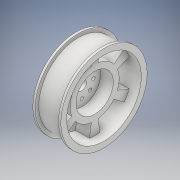
# Autodesk Inventor part: 바퀴8PI
Saved by Autodesk Inventor 2017 (Build 210142000, 142)
## iProperties
Part Number: 바퀴8PI
Material: ABS 플라스틱
Document SubType Name: Modeling
Designer: minom
Density: 1.06 g/cm^3
Appearance: 매끄러움 - 흰색
Mass: 45.626 g
Surface Area: 218.795 cm^2
Volume: 43.0434 cm^3
Author: minom
Autodesk Inventor part; units mm, degrees
ref_plane "YZ Plane" through (0, 0, 0) normal (1, 0, 0) x (0, 1, 0)
ref_plane "XZ Plane" through (0, 0, 0) normal (0, 1, 0) x (-1, 0, 0)
ref_plane "XY Plane" through (0, 0, 0) normal (0, 0, 1) x (1, 0, 0)
sketch "스케치1" plane through (0, 0, 0) normal (1, 0, 0) x (0, 1, 0)
  circle A0 centre (0, 0) radius 37
  circle A1 centre (0, 0) radius 4
  dimension "d0" = 74
  dimension "d1" = 8
  constraints: 2 centre point, 2 coincident
  measures "d0" diameter of A0
  measures "d1" diameter of A1
extrude "돌출1" add sketch "스케치1" along normal blind 24
sketch "스케치2" plane through (24, 0, 0) normal (1, 0, 0) x (0, 0, -1)
  circle A0 centre (0, 0) radius 16
  dimension "d4" = 32
  constraints: 1 centre point, 1 coincident
  measures "d4" diameter of A0
extrude "돌출2" cut sketch "스케치2" against normal blind 19
sketch "스케치4" plane through (5, 0, 0) normal (1, 0, 0) x (0, 0, -1)
  circle A0 centre (0, 10) radius 1.5
  circle A1 centre (10, 0) radius 1.5
  circle A2 centre (0, -10) radius 1.5
  circle A3 centre (-10, 0) radius 1.5
  circle A4 centre (7.0711, -7.0711) radius 1.5
  circle A5 centre (7.0711, 7.0711) radius 1.5
  circle A6 centre (-7.0711, 7.0711) radius 1.5
  circle A7 centre (-7.0711, -7.0711) radius 1.5
  point P0 (0, 0)
  dimension "d8" = 3
  dimension "d9" = 3
  dimension "d10" = 3
  dimension "d11" = 3
  dimension "d28" = 3
  dimension "d29" = 3
  dimension "d30" = 3
  dimension "d31" = 3
  constraints: 8 centre point
  measures "d8" diameter of A0
  measures "d9" diameter of A1
  measures "d10" diameter of A2
  measures "d11" diameter of A3
  measures "d28" diameter of A4
  measures "d29" diameter of A5
  measures "d30" diameter of A6
  measures "d31" diameter of A7
extrude "돌출3" cut sketch "스케치4" against normal blind 5
sketch "스케치6" plane through (24, 0, 0) normal (1, 0, 0) x (0, 0, -1)
  circle A0 centre (0, 0) radius 34
  circle A1 centre (0, 0) radius 16 projected
  circle A2 centre (0, 0) radius 37 projected
  dimension "d22" = 68
  constraints: 1 centre point, 1 coincident
  measures "d22" diameter of A0
ref_plane "작업 평면1" through (24, 0, 0) normal (1, 0, 0) x (0, 0, -1)
sketch "스케치7" plane through (24, 0, 0) normal (1, 0, 0) x (0, 0, -1)
  circle A0 centre (0, 0) radius 37
  circle A1 centre (0, 0) radius 34
  dimension "d25" = 74
  dimension "d102" = 68
  constraints: 2 centre point, 2 coincident
  measures "d25" diameter of A0
  measures "d102" diameter of A1
ref_plane "작업 평면2" through (24, 0, 0) normal (1, 0, 0) x (0, 0, -1)
sketch "스케치11" plane through (24, 0, 0) normal (1, 0, 0) x (0, 0, -1)
  circle A0 centre (0, 0) radius 16 projected
  circle A1 centre (0, 0) radius 37 projected
  line L0 (19.7012, -25.2163) -> (12.9289, -16.5482)
  line L1 (-12.9289, 16.5482) -> (-19.7012, 25.2163)
  line L2 (11.9874, -29.6699) -> (7.8667, -19.4709)
  line L3 (-7.8667, 19.4709) -> (-11.9874, 29.6699)
  line L4 (11.9874, 29.6699) -> (7.8667, 19.4709)
  line L5 (-7.8667, -19.4709) -> (-11.9874, -29.6699)
  line L6 (19.7012, 25.2163) -> (12.9289, 16.5482)
  line L7 (-12.9289, -16.5482) -> (-19.7012, -25.2163)
  line L8 (-31.6886, -4.4535) -> (-20.7956, -2.9226)
  line L9 (20.7956, 2.9226) -> (31.6886, 4.4535)
  line L10 (-31.6886, 4.4535) -> (-20.7956, 2.9226)
  line L11 (20.7956, -2.9226) -> (31.6886, -4.4535)
  arc A2 (7.8667, 19.4709) -> (-7.8667, 19.4709) centre (0, 0) ccw
  arc A3 (11.9874, 29.6699) -> (-11.9874, 29.6699) centre (0, 0) ccw
  arc A4 (31.6886, 4.4535) -> (19.7012, 25.2163) centre (0, 0) ccw
  arc A5 (20.7956, 2.9226) -> (12.9289, 16.5482) centre (0, 0) ccw
  arc A6 (12.9289, -16.5482) -> (20.7956, -2.9226) centre (0, 0) ccw
  arc A7 (19.7012, -25.2163) -> (31.6886, -4.4535) centre (0, 0) ccw
  arc A8 (-7.8667, -19.4709) -> (7.8667, -19.4709) centre (0, 0) ccw
  arc A9 (-11.9874, -29.6699) -> (11.9874, -29.6699) centre (0, 0) ccw
  arc A10 (-19.7012, 25.2163) -> (-31.6886, 4.4535) centre (0, 0) ccw
  arc A11 (-31.6886, -4.4535) -> (-19.7012, -25.2163) centre (0, 0) ccw
  arc A12 (-12.9289, 16.5482) -> (-20.7956, 2.9226) centre (0, 0) ccw
  arc A13 (-20.7956, -2.9226) -> (-12.9289, -16.5482) centre (0, 0) ccw
  constraints: 24 end point, 24 point on circle, 12 centre point
extrude "돌출12" cut sketch "스케치11" against normal blind 20 contours L0 A6 L11 A7 | A12 L10 A10 L1 | A9 L5 A8 L2 | L3 A3 L4 A2 | A4 L9 A5 L6 | L7 A11 L8 A13
extrude "돌출14" cut sketch "스케치6" against normal blind 22 contours A2
extrude "돌출15" add sketch "스케치7" against normal blind 2
sketch "스케치13" plane through (24, 0, 0) normal (1, 0, 0) x (0, 0, -1)
  circle A0 centre (0, 0) radius 37 projected
  arc A1 (20.7956, 2.9226) -> (12.9289, 16.5482) centre (0, 0) ccw projected
  line L0 (12.9289, 16.5482) -> (19.7012, 25.2163) projected
  arc A2 (31.6886, 4.4535) -> (19.7012, 25.2163) centre (0, 0) ccw projected
  line L1 (31.6886, 4.4535) -> (20.7956, 2.9226) projected
  line L2 (-7.8667, 19.4709) -> (-11.9874, 29.6699) projected
  arc A3 (11.9874, 29.6699) -> (-11.9874, 29.6699) centre (0, 0) ccw projected
  line L3 (11.9874, 29.6699) -> (7.8667, 19.4709) projected
  arc A4 (7.8667, 19.4709) -> (-7.8667, 19.4709) centre (0, 0) ccw projected
  arc A5 (12.9289, -16.5482) -> (20.7956, -2.9226) centre (0, 0) ccw projected
  line L4 (20.7956, -2.9226) -> (31.6886, -4.4535) projected
  arc A6 (19.7012, -25.2163) -> (31.6886, -4.4535) centre (0, 0) ccw projected
  line L5 (19.7012, -25.2163) -> (12.9289, -16.5482) projected
  line L6 (-20.7956, 2.9226) -> (-31.6886, 4.4535) projected
  arc A7 (-19.7012, 25.2163) -> (-31.6886, 4.4535) centre (0, 0) ccw projected
  line L7 (-19.7012, 25.2163) -> (-12.9289, 16.5482) projected
  arc A8 (-12.9289, 16.5482) -> (-20.7956, 2.9226) centre (0, 0) ccw projected
  arc A9 (-7.8667, -19.4709) -> (7.8667, -19.4709) centre (0, 0) ccw projected
  line L8 (7.8667, -19.4709) -> (11.9874, -29.6699) projected
  arc A10 (-11.9874, -29.6699) -> (11.9874, -29.6699) centre (0, 0) ccw projected
  line L9 (-11.9874, -29.6699) -> (-7.8667, -19.4709) projected
  arc A11 (-20.7956, -2.9226) -> (-12.9289, -16.5482) centre (0, 0) ccw projected
  line L10 (-12.9289, -16.5482) -> (-19.7012, -25.2163) projected
  arc A12 (-31.6886, -4.4535) -> (-19.7012, -25.2163) centre (0, 0) ccw projected
  line L11 (-31.6886, -4.4535) -> (-20.7956, -2.9226) projected
  circle A13 centre (0, 0) radius 16 projected
  circle A14 centre (0, 0) radius 32
  constraints: 1 centre point, 1 coincident
extrude "돌출16" cut sketch "스케치13" against normal blind 8 contours L1 A14 L4 A5 L5 L8 A9 L9 L10 A11 L11 L6 A8 L7 L2 A4 L3 L0 A1
